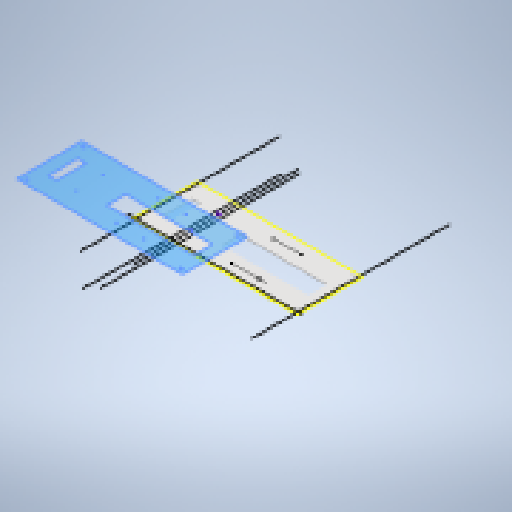
# Autodesk Inventor part: 발 받침대 받침_윗면
Saved by Autodesk Inventor 2024 (Build 280153000, 153)
## iProperties
Created: 2024-04-10
Part Number: 발 받침대 받침_윗면
Material: 일반
Document SubType Name: Modeling
Designer: ckhye
Density: 1 g/cm^3
Appearance: 기본값
Author: ckhye
Autodesk Inventor part; units mm, degrees
ref_plane "YZ Plane" through (0, 0, 0) normal (1, 0, 0) x (0, 1, 0)
ref_plane "XZ Plane" through (0, 0, 0) normal (0, 1, 0) x (-1, 0, 0)
ref_plane "XY Plane" through (0, 0, 0) normal (0, 0, 1) x (1, 0, 0)
sketch "스케치1" plane through (0, 0, 0) normal (0, 1, 0) x (-1, 0, 0)
  line L0 (195, 76.5) -> (-195, 76.5)
  line L1 (-195, 76.5) -> (-195, -76.5)
  line L2 (-195, -76.5) -> (195, -76.5)
  line L3 (195, -76.5) -> (195, 76.5)
  line L4 (195, 76.5) -> (-195, -76.5) construction
  line L5 (-195, 76.5) -> (195, -76.5) construction
  point P0 (0, 0)
  dimension "d0" = 390
  dimension "d1" = 153
  constraints: 12 end point, 2 midpoint, 2 parallel, 1 horizontal, 1 perpendicular
  measures "d0" distance of L2.end L1.end
  measures "d1" distance between parallel lines of L2 L0
extrude "돌출1" add sketch "스케치1" along normal blind 3
sketch "스케치2" plane through (0, 3, 0) normal (0, 1, 0) x (1, 0, 0)
  line L0 (-101, -167.7961) -> (-101, 220.4195)
  line L1 (-195, 76.5) -> (-195, -76.5) projected
  line L2 (-195, -76.5) -> (195, -76.5) projected
  circle A0 centre (-101, -31.5) radius 2
  circle A1 centre (-101, 33.5) radius 2
  line L3 (195, -76.5) -> (195, 76.5) projected
  line L4 (-91, -255.1075) -> (-91, 213.2428)
  line L5 (-111, -276.0921) -> (-111, 192.2583)
  line L6 (-190, -202.8267) -> (-190, 265.5236)
  line L7 (190, -180.3404) -> (190, 288.01)
  line L8 (-211.2868, -71.5) -> (199.2371, -71.5)
  circle A2 centre (12.5, -49.5) radius 2
  circle A3 centre (77.5, -49.5) radius 2
  circle A4 centre (12.5, 49.5) radius 2
  circle A5 centre (77.5, 49.5) radius 2
  line L9 (12.5, -49.5) -> (99.2818, -49.5) construction
  line L10 (12.5, 49.5) -> (77.5, 49.5) construction
  line L11 (195, 76.5) -> (-195, 76.5) projected
  dimension "d4" = 94
  dimension "d10" = 4
  dimension "d11" = 4
  dimension "d23" = 10
  dimension "d24" = 10
  dimension "d25" = 5
  dimension "d26" = 5
  dimension "d27" = 5
  dimension "d38" = 4
  dimension "d39" = 4
  dimension "d40" = 4
  dimension "d41" = 4
  dimension "d42" = 65
  dimension "d43" = 65
  dimension "d44" = 117.5
  dimension "d45" = 117.5
  dimension "d46" = 27
  dimension "d47" = 27
  constraints: 16 end point, 6 centre point, 5 vertical, 3 horizontal, 3 point on line
  measures "d4" distance between parallel lines of L0 L1
  measures "d10" diameter of A0
  measures "d11" diameter of A1
  measures "d23" distance between parallel lines of L0 L4
  measures "d24" distance between parallel lines of L0 L5
  measures "d25" distance between parallel lines of L3 L7
  measures "d26" distance between parallel lines of L1 L6
  measures "d27" distance between parallel lines of L2 L8
  measures "d38" diameter of A5
  measures "d39" diameter of A3
  measures "d40" diameter of A2
  measures "d41" diameter of A4
  measures "d42" distance of L10.end L10.start
  measures "d43" distance of A3.centre L9.start
  measures "d44" distance from line of L3 A3.centre
  measures "d45" distance from line of L10.end L3
  measures "d46" distance from line of L2 A3.centre
  measures "d47" distance from line of L11 L10.end
extrude "돌출2" cut sketch "스케치2" against normal up to surface (3 mm away) contours A0 L0 | L0 A0 | A1 L0 | L0 A1 | A2 | A3 | A4 | A5
sketch "스케치3" plane through (0, 0, 0) normal (0, -1, 0) x (1, 0, 0)
  line L0 (-35, 25) -> (170, 25)
  line L1 (170, 25) -> (170, -20)
  line L2 (170, -20) -> (-35, -20)
  line L3 (-35, -20) -> (-35, 25)
  line L4 (-35, 25) -> (170, -20) construction
  line L5 (170, 25) -> (-35, -20) construction
  line L6 (195, 76.5) -> (195, -76.5) projected
  line L7 (-165, 33.5) -> (-145, 33.5)
  line L8 (-145, 33.5) -> (-145, -36.5)
  line L9 (-145, -36.5) -> (-165, -36.5)
  line L10 (-165, -36.5) -> (-165, 33.5)
  line L11 (195, -76.5) -> (-195, -76.5) projected
  line L12 (-195, -76.5) -> (-195, 76.5) projected
  point P0 (0, 0)
  point P1 (67.5, 2.5)
  dimension "d28" = 205
  dimension "d29" = 25
  dimension "d30" = 45
  dimension "d31" = 20
  dimension "d34" = 70
  dimension "d35" = 20
  dimension "d36" = 110
  dimension "d37" = 30
  constraints: 20 end point, 4 parallel, 2 horizontal, 2 midpoint, 2 perpendicular
  measures "d28" distance of L1.end L2.end
  measures "d29" distance between parallel lines of L6 L1
  measures "d30" distance of L0.end L1.end
  measures "d31" distance from line of point (0, 0) L2
  measures "d34" distance of L9.end L7.start
  measures "d35" distance of L7.start L7.end
  measures "d36" distance between parallel lines of L11 L7
  measures "d37" distance between parallel lines of L12 L10
extrude "돌출3" cut sketch "스케치3" against normal blind 10
sketch "스케치6" plane through (0, 0, 0) normal (0, -1, 0) x (1, 0, 0)
  line L0 (-184, -66.5) -> (-180, -66.5) construction
  line L1 (-184, -68.5) -> (-180, -68.5)
  line L2 (-180, -64.5) -> (-184, -64.5)
  arc A0 (-184, -64.5) -> (-184, -68.5) centre (-184, -66.5) ccw
  arc A1 (-180, -68.5) -> (-180, -64.5) centre (-180, -66.5) ccw
  line L3 (-195, -76.5) -> (-195, 76.5) projected
  line L4 (195, -76.5) -> (-195, -76.5) projected
  line L5 (0, -8.9008) -> (0, 5.7448)
  line L6 (-2.4122, 0) -> (4.9846, 0)
  line L7 (184, -66.5) -> (180, -66.5) construction
  line L8 (184, -68.5) -> (180, -68.5)
  line L9 (180, -64.5) -> (184, -64.5)
  arc A2 (184, -68.5) -> (184, -64.5) centre (184, -66.5) ccw
  arc A3 (180, -64.5) -> (180, -68.5) centre (180, -66.5) ccw
  line L10 (-184, 66.5) -> (-180, 66.5) construction
  line L11 (-184, 68.5) -> (-180, 68.5)
  line L12 (-180, 64.5) -> (-184, 64.5)
  arc A4 (-184, 68.5) -> (-184, 64.5) centre (-184, 66.5) ccw
  arc A5 (-180, 64.5) -> (-180, 68.5) centre (-180, 66.5) ccw
  line L13 (184, 66.5) -> (180, 66.5) construction
  line L14 (184, 68.5) -> (180, 68.5)
  line L15 (180, 64.5) -> (184, 64.5)
  arc A6 (184, 64.5) -> (184, 68.5) centre (184, 66.5) ccw
  arc A7 (180, 68.5) -> (180, 64.5) centre (180, 66.5) ccw
  point P0 (0, 0)
  point P1 (-182, -66.5)
  point P2 (182, -66.5)
  point P3 (-182, 66.5)
  point P4 (182, 66.5)
  dimension "d87" = 4
  dimension "d88" = 4
  dimension "d89" = 13
  dimension "d90" = 10
  constraints: 36 end point, 21 symmetric about line, 16 point on circle, 8 centre point, 4 tangent, 2 horizontal, 1 midpoint, 1 parallel, 1 vertical, 6 other
  measures "d87" distance of L0.start L0.end
  measures "d88" diameter of A1
  measures "d89" distance from line of L3 point (-182, -66.5)
  measures "d90" distance from line of L4 point (-182, -66.5)
extrude "돌출5" cut sketch "스케치6" against normal blind 10
equation "\"d45\" = d44"
equation "\"d47\" = d46"
